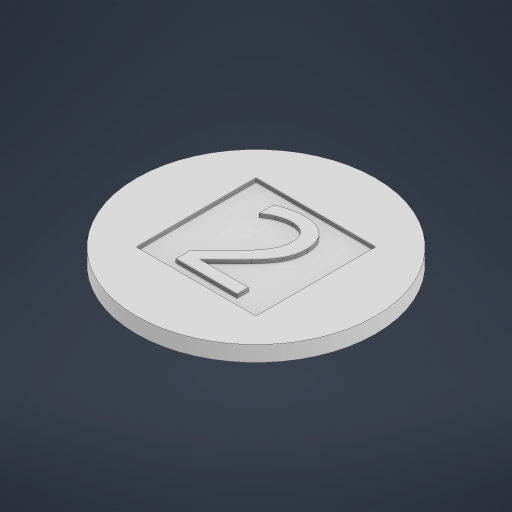
# Autodesk Inventor part: TopMarker2
Saved by Autodesk Inventor 2023 (Build 270158000, 158)
## iProperties
Created: 2023-03-04
Part Number: TopMarker2
Material: Generic
Document SubType Name: Modeling
Designer: Elias Braun
Density: 1 g/cm^3
Appearance: Default
Author: Elias Braun
Autodesk Inventor part; units mm, degrees
ref_plane "YZ Plane" through (0, 0, 0) normal (1, 0, 0) x (0, 1, 0)
ref_plane "XZ Plane" through (0, 0, 0) normal (0, 1, 0) x (-1, 0, 0)
ref_plane "XY Plane" through (0, 0, 0) normal (0, 0, 1) x (1, 0, 0)
sketch "Sketch1" plane through (0, 0, 0) normal (0, 1, 0) x (-1, 0, 0)
  circle A0 centre (0, 0) radius 20
  dimension "d0" = 40
  constraints: 1 centre point, 1 coincident
  measures "d0" diameter of A0
extrude "Extrusion1" add sketch "Sketch1" along normal blind 2.6
sketch "Sketch2" plane through (0, 2.6, 0) normal (0, 1, 0) x (1, 0, 0)
  line L0 (-10, -10) -> (10, -10)
  line L1 (10, -10) -> (10, 10)
  line L2 (10, 10) -> (-10, 10)
  line L3 (-10, 10) -> (-10, -10)
  line L4 (-10, -10) -> (10, 10) construction
  line L5 (10, -10) -> (-10, 10) construction
  point P0 (0, 0)
  dimension "d3" = 20
  dimension "d4" = 20
  constraints: 12 end point, 2 midpoint, 2 parallel, 1 horizontal, 1 perpendicular
  measures "d3" distance of L0.start L0.end
  measures "d4" distance of L1.end L0.end
extrude "Extrusion2" cut sketch "Sketch2" against normal blind 0.6
sketch "Sketch3" plane through (0, 2, 0) normal (0, 1, 0) x (1, 0, 0)
  line L0 (-6.2058, 8.5439) -> (6.2509, 8.5439) construction
  line L1 (6.2509, 8.5439) -> (6.2509, -8.4059) construction
  line L2 (6.2509, -8.4059) -> (-6.2058, -8.4059) construction
  line L3 (-6.2058, -8.4059) -> (-6.2058, 8.5439) construction
  line L4 (5.242, -8.4059) -> (-4.9952, -8.4059)
  line L5 (-4.9952, -8.4059) -> (-4.9952, -6.0518)
  spline S0 degree 2 poles (-4.9952, -6.0518) (-3.8921, -5.0159) (-1.9281, -3.0923) (-0.9864, -2.0565) knots 0 0 0 1 2 2 2
  spline S1 degree 2 poles (-0.9864, -2.0565) (0.9104, 0.0286) (2.2959, 2.5307) (2.2959, 3.8625) knots 0 0 0 1 2 2 2
  spline S2 degree 2 poles (2.2959, 3.8625) (2.2959, 4.562) (1.8655, 5.6113) (1.4754, 5.9476) knots 0 0 0 1 2 2 2
  spline S3 degree 2 poles (1.4754, 5.9476) (1.0852, 6.2839) (0.0629, 6.6202) (-0.5559, 6.6202) knots 0 0 0 1 2 2 2
  spline S4 degree 2 poles (-0.5559, 6.6202) (-1.1478, 6.6202) (-2.3585, 6.3243) (-2.9101, 6.0956) knots 0 0 0 1 2 2 2
  spline S5 degree 2 poles (-2.9101, 6.0956) (-3.3809, 5.9072) (-4.2553, 5.3691) (-4.5243, 5.1808) knots 0 0 0 1 2 2 2
  line L6 (-4.5243, 5.1808) -> (-4.6454, 5.1808)
  line L7 (-4.6454, 5.1808) -> (-4.6454, 7.5484)
  spline S6 degree 2 poles (-4.6454, 7.5484) (-3.9593, 7.8847) (-1.4976, 8.5439) (-0.3945, 8.5439) knots 0 0 0 1 2 2 2
  spline S7 degree 2 poles (-0.3945, 8.5439) (1.9327, 8.5439) (4.5559, 6.0821) (4.5559, 3.9836) knots 0 0 0 1 2 2 2
  spline S8 degree 2 poles (4.5559, 3.9836) (4.5559, 3.0016) (4.0985, 1.3604) (3.695, 0.6609) knots 0 0 0 1 2 2 2
  spline S9 degree 2 poles (3.695, 0.6609) (3.2914, -0.0655) (2.1211, -1.4915) (1.4754, -2.1775) knots 0 0 0 1 2 2 2
  spline S10 degree 2 poles (1.4754, -2.1775) (0.4261, -3.321) (-2.1433, -5.7693) (-2.9101, -6.4822) knots 0 0 0 1 2 2 2
  line L8 (-2.9101, -6.4822) -> (5.242, -6.4822)
  line L9 (5.242, -6.4822) -> (5.242, -8.4059)
  point P0 (0, 0)
  constraints: 2 other
extrude "Extrusion3" add sketch "Sketch3" along normal blind 0.6
body "Solid1"
